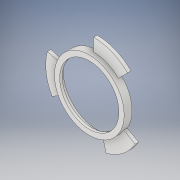
# Autodesk Inventor part: FanMount
Saved by Autodesk Inventor 2017 (Build 210142000, 142)
## iProperties
Created: 2016-04-16
Part Number: FanMount
Material: PC/ABS Plastic
Document SubType Name: Modeling
Designer: jbreeden
Density: 0.357273 g/cm^3
Appearance: Smooth - White
Author: jbreeden
Autodesk Inventor part; units mm, degrees
ref_plane "YZ Plane" through (0, 0, 0) normal (1, 0, 0) x (0, 1, 0)
ref_plane "XZ Plane" through (0, 0, 0) normal (0, 1, 0) x (-1, 0, 0)
ref_plane "XY Plane" through (0, 0, 0) normal (0, 0, 1) x (1, 0, 0)
sketch "Sketch1" plane through (0, 0, 0) normal (0, 1, 0) x (-1, 0, 0)
  line L0 (0, 0) -> (21.717, 0)
  line L1 (0, 0) -> (0, -12.7)
  line L2 (21.717, 0) -> (24.765, 0)
  line L3 (24.765, 0) -> (24.765, -3.81)
  line L4 (24.765, -3.81) -> (21.717, 0)
  line L5 (24.765, 0) -> (25.4, 0)
  line L6 (25.4, 0) -> (25.4, -3.81)
  line L7 (25.4, -3.81) -> (24.765, -3.81)
  line L8 (24.765, -3.81) -> (24.765, 0)
  line L9 (25.4, 0) -> (21.59, 0)
  line L10 (21.59, 0) -> (21.59, 1.905)
  line L11 (21.59, 1.905) -> (25.4, 1.905)
  line L12 (25.4, 1.905) -> (25.4, 0)
  dimension "d0" = 21.717
  dimension "d1" = 12.7
  dimension "d2" = 3.048
  dimension "d3" = 3.81
  dimension "d4" = 0.635
  dimension "d6" = 1.905
  constraints: 26 end point, 4 horizontal, 4 parallel, 2 perpendicular, 2 vertical
  measures "d0" distance of L0.start L0.end
  measures "d1" distance of L0.start L1.end
  measures "d2" distance of L0.end L2.end
  measures "d3" distance of L2.end L3.end
  measures "d4" distance of L6.end L7.end
  measures "d6" distance of L9.end L10.end
revolve "Revolution1" add sketch "Sketch1" angle 360 about axis through (0, 0, 0) along (0, 0, -1)
sketch "Sketch3" plane through (0, 0, -3.81) normal (0, 0, -1) x (-1, 0, 0)
  circle A0 centre (0, 0) radius 25.4
  circle A1 centre (0, 0) radius 34.925
  line L0 (0, 0) -> (0, 34.925)
  line L1 (0, 0) -> (-24.6957, 24.6957)
  line L2 (0, 0) -> (34.925, 0) construction
  circle A2 centre (0, 0) radius 25.4 projected
  line L3 (0, 0) -> (-30.2459, -17.4625)
  line L4 (0, 0) -> (34.925, 0) construction
  line L5 (0, 0) -> (-9.0393, -33.735)
  line L6 (0, 0) -> (34.925, 0) construction
  line L7 (0, 0) -> (30.2459, -17.4625)
  line L8 (0, 0) -> (34.925, 0) construction
  line L9 (0, 0) -> (33.735, 9.0393)
  line L10 (0, 0) -> (34.925, 0) construction
  arc A3 (0, 25.4) -> (-17.9605, 17.9605) centre (0, 0) ccw
  arc A4 (-21.997, -12.7) -> (-6.574, -24.5345) centre (0, 0) ccw
  arc A5 (21.997, -12.7) -> (24.5345, 6.574) centre (0, 0) ccw
  dimension "d7" = 69.85
  dimension "d8" = 135
  dimension "d9" = 150
  dimension "d10" = 105
  dimension "d11" = 30
  dimension "d12" = 15
  constraints: 22 end point, 18 point on circle, 6 point on line, 5 centre point, 5 equal length, 5 horizontal, 2 coincident, 1 vertical
  measures "d7" diameter of A1
  measures "d8" angle of L2 L1
  measures "d9" angle of L3 L4
  measures "d10" angle of L5 L6
  measures "d11" angle of L7 L8
  measures "d12" angle of L10 L9
extrude "Extrusion1" add sketch "Sketch3" against normal blind 2.54 contours A0 L9 A1 L7 | A0 L1 A1 L0 | L5 A1 L3 A0
body "Solid1"
